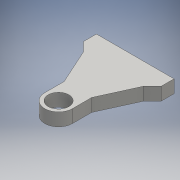
# Autodesk Inventor part: Wheel Holder
Saved by Autodesk Inventor 2016 (Build 200138000, 138)
## iProperties
Created: 2016-02-23
Part Number: Wheel Holder
Material: Generic
Document SubType Name: Modeling
Designer: Kenneth Daniel
Density: 1 g/cm^3
Appearance: Default
Author: Kenneth Daniel
Autodesk Inventor part; units mm, degrees
ref_plane "YZ Plane" through (0, 0, 0) normal (1, 0, 0) x (0, 1, 0)
ref_plane "XZ Plane" through (0, 0, 0) normal (0, 1, 0) x (-1, 0, 0)
ref_plane "XY Plane" through (0, 0, 0) normal (0, 0, 1) x (1, 0, 0)
sketch "Sketch1" plane through (0, 0, 0) normal (0, 0, 1) x (1, 0, 0)
  line L0 (0, 0) -> (60, 0)
  line L1 (60, 0) -> (60, 70)
  line L2 (60, 70) -> (0, 70)
  line L3 (0, 70) -> (0, 0)
  dimension "d0" = 60
  dimension "d1" = 70
  constraints: 8 end point, 2 parallel, 1 horizontal, 1 perpendicular
  measures "d0" distance of L0.start L0.end
  measures "d1" distance of L1.end L0.end
extrude "Extrusion1" add sketch "Sketch1" along normal blind 10
sketch "Sketch2" plane through (0, 0, 10) normal (0, 0, 1) x (1, 0, 0)
  line L0 (0, 60) -> (60, 60) construction
  line L1 (60, 0) -> (60, 70) construction
  line L2 (0, 60) -> (60, 0) construction
  line L3 (0, 0) -> (60, 0) construction
  line L4 (60, 60) -> (0, 0) construction
  arc A0 (0, 0) -> (0, 60) centre (-23.1222, 30) ccw construction
  arc A1 (60, 60) -> (60, 0) centre (83.1222, 30) ccw construction
  line L5 (60, 70) -> (0, 70) construction
  line L6 (30, 70) -> (30, 0) construction
  line L7 (17.3619, 30) -> (14.7544, 30) construction
  line L8 (42.6381, 30) -> (45.2456, 30) construction
  line L9 (0, 60) -> (60, 60)
  circle A2 centre (30, 10.6788) radius 10.6788
  line L10 (19.3212, 10.6788) -> (19.3212, 25.6788)
  line L11 (6.8778, 53.1222) -> (0, 60)
  line L12 (40.6788, 10.6788) -> (40.6788, 25.6788)
  line L13 (60, 60) -> (53.1222, 53.1222)
  line L14 (6.8778, 53.1222) -> (19.3212, 25.6788)
  line L15 (53.1222, 53.1222) -> (40.6788, 25.6788)
  line L16 (0, 70) -> (0, 0) projected
  line L17 (0, 60) -> (0, 70)
  line L18 (0, 70) -> (60, 70)
  line L19 (60, 70) -> (60, 60)
  line L20 (40.6788, 25.6788) -> (19.3212, 25.6788)
  line L21 (53.1222, 53.1222) -> (6.8778, 53.1222)
  line L22 (6.8778, 53.1222) -> (0, 60)
  line L23 (53.1222, 53.1222) -> (60, 60)
  line L24 (0, 70) -> (0, 0) projected
  line L25 (0, 60) -> (0, 70)
  line L26 (0, 70) -> (60, 70)
  line L27 (60, 60) -> (60, 70)
  dimension "d4" = 10
  constraints: 46 end point, 12 point on circle, 6 point on line, 5 perpendicular, 4 collinear, 3 centre point, 2 midpoint, 2 parallel, 2 tangent, 1 horizontal
  measures "d4" distance of L0.end L1.end
extrude "Extrusion2" add sketch "Sketch2" along normal blind 10
sketch "Sketch3" plane through (60, 0, 0) normal (1, 0, 0) x (0, 0, -1)
  line L0 (-10, 60) -> (-20, 60) projected
  line L1 (-10, 60) -> (-10, 70)
  line L2 (0, 70) -> (-20, 70) projected
  line L3 (0, 0) -> (-10, 0) projected
  line L4 (-10, 0) -> (0, 0)
  line L5 (-10, 60) -> (-10, 0)
  line L6 (-10, 0) -> (-10, 60) projected
  line L7 (0, 0) -> (0, 70) projected
  line L8 (-10, 0) -> (0, 0)
  line L9 (0, 0) -> (0, 70)
  line L10 (0, 70) -> (-10, 70)
  constraints: 12 end point, 2 collinear, 2 perpendicular, 1 horizontal, 1 midpoint
extrude "Extrusion3" cut sketch "Sketch3" against normal through all
sketch "Sketch4" plane through (0, 0, 20) normal (0, 0, 1) x (1, 0, 0)
  arc A0 (19.3212, 10.6788) -> (40.6788, 10.6788) centre (30, 10.6788) ccw construction
  line L0 (30, 10.6788) -> (30, 0) construction
  line L1 (60, 70) -> (0, 70) construction
  line L2 (30, 70) -> (30, 10.6788) construction
  circle A1 centre (30, 10.6788) radius 7.9826 construction
  circle A2 centre (30, 10.6788) radius 7.9826
  point P0 (0, 0)
  constraints: 4 end point, 2 centre point, 2 coincident, 1 concentric, 1 midpoint, 1 perpendicular, 1 point on circle, 1 vertical
extrude "Extrusion4" cut sketch "Sketch4" against normal blind 10
body "Solid1"
